Autodesk Fusion 360 part; units mm, degrees
(part 2 of 2)
sketch "Sketch6" plane through (0, 0, 2) normal (0, 0, 1) x (-1, 0, 0)
  arc A0 (71.2, 43.75) -> (67.2, 47.75) centre (67.2, 43.75) ccw
  line L0 (67.2, 47.75) -> (-67.2, 47.75)
  arc A1 (-67.2, 47.75) -> (-71.2, 43.75) centre (-67.2, 43.75) ccw
  line L1 (-71.2, 43.75) -> (-71.2, -43.75)
  arc A2 (-71.2, -43.75) -> (-67.2, -47.75) centre (-67.2, -43.75) ccw
  line L2 (-67.2, -47.75) -> (67.2, -47.75)
  arc A3 (67.2, -47.75) -> (71.2, -43.75) centre (67.2, -43.75) ccw
  line L3 (71.2, -43.75) -> (71.2, 43.75)
  arc A4 (60.9079, -41.3399) -> (62.4799, -39.7679) centre (60.9079, -39.7679) ccw construction
  arc A5 (-62.4799, -39.7399) -> (-60.9079, -41.3119) centre (-60.9079, -39.7399) ccw construction
  line L4 (-48.9575, -41.8399) -> (48.9575, -41.8399) construction
  line L5 (48.9575, 41.8399) -> (-48.9575, 41.8399) construction
  line L6 (-62.9799, 29.7119) -> (-62.9799, 27.8175) construction
  line L7 (48.9575, -41.8399) -> (50.8519, -41.8399) construction
  line L8 (62.4799, 30.3078) -> (62.4799, 39.7679) construction
  arc A6 (-60.88, 42.74) -> (-63.88, 39.74) centre (-60.88, 39.74) ccw construction
  line L9 (63.88, 39.74) -> (63.88, -39.74) construction
  arc A7 (63.88, 39.74) -> (60.88, 42.74) centre (60.88, 39.74) ccw construction
  line L10 (-62.9799, -29.7119) -> (-62.4799, -30.3078) construction
  line L11 (51.4478, 41.3399) -> (50.8519, 41.8399) construction
  arc A8 (60.88, -42.74) -> (63.88, -39.74) centre (60.88, -39.74) ccw construction
  line L12 (-48.9575, 41.8399) -> (-50.8519, 41.8399) construction
  line L13 (-60.88, 42.74) -> (60.88, 42.74) construction
  line L14 (-62.9799, -27.8175) -> (-62.9799, -29.7119) construction
  line L15 (60.88, -42.74) -> (-60.88, -42.74) construction
  line L16 (62.9799, 29.7119) -> (62.4799, 30.3078) construction
  line L17 (-50.8519, 41.8399) -> (-51.4811, 41.3119) construction
  line L18 (62.4799, -39.7679) -> (62.4799, -30.3078) construction
  line L19 (-50.8519, -41.8399) -> (-48.9575, -41.8399) construction
  line L20 (60.9079, 41.3399) -> (51.4478, 41.3399) construction
  line L21 (50.8519, 41.8399) -> (48.9575, 41.8399) construction
  line L22 (62.9799, 27.8175) -> (62.9799, 29.7119) construction
  line L23 (51.4478, -41.3399) -> (60.9079, -41.3399) construction
  line L24 (62.9799, -27.8175) -> (62.9799, 27.8175) construction
  line L25 (-63.88, -39.74) -> (-63.88, 39.74) construction
  line L26 (50.8519, -41.8399) -> (51.4478, -41.3399) construction
  line L27 (62.9799, -29.7119) -> (62.9799, -27.8175) construction
  arc A9 (-63.88, -39.74) -> (-60.88, -42.74) centre (-60.88, -39.74) ccw construction
  arc A10 (62.4799, 39.7679) -> (60.9079, 41.3399) centre (60.9079, 39.7679) ccw construction
  line L28 (62.4799, -30.3078) -> (62.9799, -29.7119) construction
  line L29 (-62.4799, 30.3078) -> (-62.9799, 29.7119) construction
  line L30 (-60.9079, -41.3119) -> (-51.4811, -41.3119) construction
  arc A11 (-60.9079, 41.3119) -> (-62.4799, 39.7399) centre (-60.9079, 39.7399) ccw construction
  line L31 (-51.4811, -41.3119) -> (-50.8519, -41.8399) construction
  line L32 (-51.4811, 41.3119) -> (-60.9079, 41.3119) construction
  line L33 (-62.4799, 39.7399) -> (-62.4799, 30.3078) construction
  line L34 (-62.4799, -30.3078) -> (-62.4799, -39.7399) construction
  line L35 (-62.9799, 27.8175) -> (-62.9799, -27.8175) construction
  line L36 (0, -47.75) -> (0, 47.75) construction
  line L37 (-71.2, 0) -> (71.2, 0) construction
  line L38 (-60.85, 43.25) -> (60.85, 43.25)
  line L39 (64.35, 39.75) -> (64.35, -39.75)
  line L40 (60.85, -43.25) -> (-60.85, -43.25)
  line L41 (-64.35, -39.75) -> (-64.35, 39.75)
  line L42 (-64.35, 43.25) -> (64.35, -43.25) construction
  line L43 (64.35, 43.25) -> (-64.35, -43.25) construction
  arc A12 (60.85, -43.25) -> (64.35, -39.75) centre (60.85, -39.75) ccw
  arc A13 (-64.35, -39.75) -> (-60.85, -43.25) centre (-60.85, -39.75) ccw
  arc A14 (-60.85, 43.25) -> (-64.35, 39.75) centre (-60.85, 39.75) ccw
  arc A15 (64.35, 39.75) -> (60.85, 43.25) centre (60.85, 39.75) ccw
  line L44 (-60.85, 40.75) -> (60.85, 40.75)
  line L45 (61.85, 39.75) -> (61.85, -39.75)
  line L46 (60.85, -40.75) -> (-60.85, -40.75)
  line L47 (-61.85, -39.75) -> (-61.85, 39.75)
  line L48 (-61.85, 40.75) -> (61.85, -40.75) construction
  line L49 (61.85, 40.75) -> (-61.85, -40.75) construction
  arc A16 (-61.85, -39.75) -> (-60.85, -40.75) centre (-60.85, -39.75) ccw
  arc A17 (60.85, -40.75) -> (61.85, -39.75) centre (60.85, -39.75) ccw
  arc A18 (61.85, 39.75) -> (60.85, 40.75) centre (60.85, 39.75) ccw
  arc A19 (-60.85, 40.75) -> (-61.85, 39.75) centre (-60.85, 39.75) ccw
  dimension "d56" = 128.7
  dimension "d57" = 86.5
  dimension "d58" = 3.5
  dimension "d59" = 3.5
  dimension "d60" = 3.5
  dimension "d61" = 3.5
  dimension "d63" = 2.5
  dimension "d64" = 2.5
  dimension "d65" = 1
  dimension "d66" = 1
  dimension "d67" = 1
  dimension "d68" = 1
  constraint midpoint L2 L36.start
  constraint midpoint L0 L36.end
  constraint midpoint L1 L37.start
  constraint midpoint L3 L37.end
  constraint horizontal L38
  constraint perpendicular L38 L39
  constraint parallel L38 L40
  constraint parallel L39 L41
  constraint coincident L42 origin
  constraint coincident L43 origin
  constraint coincident L42.end L40
  constraint coincident L42.end L39
  constraint tangent L40 A12
  constraint tangent L39 A12
  constraint coincident L43.end L41
  constraint coincident L43.end L40
  constraint tangent L41 A13
  constraint tangent L40 A13
  constraint coincident L42.start L41
  constraint coincident L42.start L38
  constraint tangent L41 A14
  constraint tangent L38 A14
  constraint coincident L43.start L38
  constraint coincident L43.start L39
  constraint tangent L38 A15
  constraint tangent L39 A15
  constraint horizontal L44
  constraint perpendicular L44 L45
  constraint parallel L44 L46
  constraint parallel L45 L47
  constraint coincident L48 origin
  constraint coincident L49 origin
  constraint coincident L49.end L47
  constraint coincident L49.end L46
  constraint tangent L47 A16
  constraint tangent L46 A16
  constraint coincident L48.end L46
  constraint coincident L48.end L45
  constraint tangent L46 A17
  constraint tangent L45 A17
  constraint coincident L49.start L44
  constraint coincident L49.start L45
  constraint tangent L44 A18
  constraint tangent L45 A18
  constraint coincident L48.start L47
  constraint coincident L48.start L44
  constraint tangent L47 A19
  constraint tangent L44 A19
  measures "d56" distance of L42.end L43.end
  measures "d57" distance of L43.start L42.end
  measures "d58" radius of A12
  measures "d59" radius of A13
  measures "d60" radius of A14
  measures "d61" radius of A15
  measures "d63" distance of L41 L47
  measures "d64" distance of L40 L46
  measures "d65" radius of A16
  measures "d66" radius of A17
  measures "d67" radius of A18
  measures "d68" radius of A19
extrude "Extrude7" cut sketch "Sketch6" against normal blind 1 contours L38 L39 L40 L41 A12 A13 A14 A15
sketch "Sketch4" plane through (0, 0, 2) normal (0, 0, 1) x (-1, 0, 0)
  line L0 (-67.2, -47.75) -> (67.2, -47.75)
  line L1 (71.2, -43.75) -> (71.2, 43.75)
  line L2 (67.2, 47.75) -> (-67.2, 47.75)
  line L3 (-71.2, 43.75) -> (-71.2, -43.75)
  line L4 (-52.85, 35.75) -> (52.85, 35.75)
  line L5 (56.85, 31.75) -> (56.85, -31.75)
  line L6 (52.85, -35.75) -> (-52.85, -35.75)
  line L7 (-56.85, -31.75) -> (-56.85, 31.75)
  line L8 (-56.85, 35.75) -> (56.85, -35.75) construction
  line L9 (56.85, 35.75) -> (-56.85, -35.75) construction
  arc A0 (71.2, 43.75) -> (67.2, 47.75) centre (67.2, 43.75) ccw
  arc A1 (-67.2, 47.75) -> (-71.2, 43.75) centre (-67.2, 43.75) ccw
  arc A2 (-71.2, -43.75) -> (-67.2, -47.75) centre (-67.2, -43.75) ccw
  arc A3 (67.2, -47.75) -> (71.2, -43.75) centre (67.2, -43.75) ccw
  arc A4 (52.85, -35.75) -> (56.85, -31.75) centre (52.85, -31.75) ccw
  arc A5 (-56.85, -31.75) -> (-52.85, -35.75) centre (-52.85, -31.75) ccw
  arc A6 (-52.85, 35.75) -> (-56.85, 31.75) centre (-52.85, 31.75) ccw
  arc A7 (56.85, 31.75) -> (52.85, 35.75) centre (52.85, 31.75) ccw
  line L10 (64.35, 39.75) -> (64.35, -39.75)
  arc A8 (60.85, -43.25) -> (64.35, -39.75) centre (60.85, -39.75) ccw
  line L11 (60.85, -43.25) -> (-60.85, -43.25)
  arc A9 (-64.35, -39.75) -> (-60.85, -43.25) centre (-60.85, -39.75) ccw
  line L12 (-64.35, -39.75) -> (-64.35, 39.75)
  arc A10 (-60.85, 43.25) -> (-64.35, 39.75) centre (-60.85, 39.75) ccw
  line L13 (-60.85, 43.25) -> (60.85, 43.25)
  arc A11 (64.35, 39.75) -> (60.85, 43.25) centre (60.85, 39.75) ccw
  line L14 (61.85, -39.75) -> (61.85, 39.75)
  arc A12 (61.85, 39.75) -> (60.85, 40.75) centre (60.85, 39.75) ccw
  line L15 (60.85, 40.75) -> (-60.85, 40.75)
  arc A13 (-60.85, 40.75) -> (-61.85, 39.75) centre (-60.85, 39.75) ccw
  line L16 (-61.85, 39.75) -> (-61.85, -39.75)
  arc A14 (-61.85, -39.75) -> (-60.85, -40.75) centre (-60.85, -39.75) ccw
  line L17 (-60.85, -40.75) -> (60.85, -40.75)
  arc A15 (60.85, -40.75) -> (61.85, -39.75) centre (60.85, -39.75) ccw
  dimension "d71" = 4
  dimension "d72" = 4
  dimension "d73" = 4
  dimension "d74" = 4
  dimension "d77" = 5
  dimension "d78" = 5
  constraint horizontal L4
  constraint perpendicular L4 L5
  constraint parallel L4 L6
  constraint parallel L5 L7
  constraint coincident L8 origin
  constraint coincident L9 origin
  constraint coincident L8.end L6
  constraint coincident L8.end L5
  constraint tangent L6 A4
  constraint tangent L5 A4
  constraint coincident L9.end L6
  constraint coincident L9.end L7
  constraint tangent L6 A5
  constraint tangent L7 A5
  constraint coincident L8.start L7
  constraint coincident L8.start L4
  constraint tangent L7 A6
  constraint tangent L4 A6
  constraint coincident L9.start L4
  constraint coincident L9.start L5
  constraint tangent L4 A7
  constraint tangent L5 A7
  measures "d71" radius of A4
  measures "d72" radius of A5
  measures "d73" radius of A6
  measures "d74" radius of A7
  measures "d77" distance of L7 L16
  measures "d78" distance of L6 L17
extrude "Extrude8" cut sketch "Sketch4" against normal blind 5 contours L4 L5 L6 L7 A4 A5 A6 A7
equation "d9 = ( ORingPerimeter - 100 mm ) / 4 + 50 mm"
equation "ORingDiameter = 1.78 mm" comment "Diamter of the O ring"
equation "ORingInnerDiameter = 170 mm" comment "Inner diamter of the o ring bore"
equation "ORingPerimeter = 2 * 3.1412 * ( ( ORingInnerDiameter / 2 ) + ORingDiameter / 2 )"
equation "PanelWidth = 80 mm"
equation "PanelLength = 115 mm"
equation "d15 = ( ORingPerimeter - 100 mm ) / 4"
equation "d16 = ( ( ORingDiameter * 1.05 ) / 2 ) + 1.2 mm"
equation "d17 = ( ( ORingDiameter * 1.05 ) / 2 ) + 1.2 mm"
equation "d18 = ( ( ORingDiameter * 1.05 ) / 2 ) + 1.2 mm"
equation "d19 = ( ( ORingDiameter * 1.05 ) / 2 ) + 1.2 mm"
equation "d20 = ( ORingDiameter ) * 6 + ORingDiameter * 0.05 - 1.2 mm"
equation "d21 = ( ORingDiameter ) * 6 + ( ORingDiameter * 1.1 ) + 1.2 mm"
equation "d22 = -ORingDiameter * 0.8"
equation "d30 = Insert_OD - 0.5 mm"
equation "ORing2Diameter = 2 mm" comment "Second O ring Diameter"
equation "ORing2InnerDiameter = 126 mm" comment "Inner diameter of the second O Ring"
equation "ORing2Perimeter = 2 * 3.1412 * ( ( ORing2InnerDiameter / 2 ) + ORing2Diameter / 2 )"
equation "Bolt_Diam = 4 mm" comment "Diameter of the bolt"
equation "Bolt_Head_Height = 4 mm" comment "height of the bolt head"
equation "Bolt_Head_Diam = 7.22 mm" comment "Diameter of the bolt head"
equation "Insert_OD = 5.7 mm" comment "Outer Diameter of the insert"
